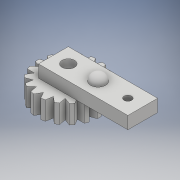
# Autodesk Inventor part: Parcial3
Saved by Autodesk Inventor 2018 (Build 220112000, 112)
## iProperties
Created: 2020-06-26
Part Number: Parcial3
Material: Generic
Document SubType Name: Modeling
Designer: Ivan
Density: 1 g/cm^3
Appearance: Default
Author: Ivan
Autodesk Inventor part; units mm, degrees
ref_plane "YZ Plane" through (0, 0, 0) normal (1, 0, 0) x (0, 1, 0)
ref_plane "XZ Plane" through (0, 0, 0) normal (0, 1, 0) x (-1, 0, 0)
ref_plane "XY Plane" through (0, 0, 0) normal (0, 0, 1) x (1, 0, 0)
sketch "Sketch1" plane through (0, 0, 0) normal (0, 0, 1) x (1, 0, 0)
  circle A0 centre (0, 0) radius 25
  circle A1 centre (0, 0) radius 5
  dimension "d0" = 50
  dimension "d1" = 10
  constraints: 2 centre point, 2 coincident
  measures "d0" diameter of A0
  measures "d1" diameter of A1
extrude "Extrusion1" add sketch "Sketch1" along normal blind 15
sketch "Sketch2" plane through (0, 0, 15) normal (0, 0, 1) x (1, 0, 0)
  circle A0 centre (0, 0) radius 25 projected
  line L0 (0, 25) -> (5, 25) construction
  line L1 (0, 20) -> (2.7962, 24.8431)
  line L2 (0, 20) -> (6.1776, 20) construction
  line L3 (0, 20) -> (-2.7962, 24.8431)
  arc A1 (2.7962, 24.8431) -> (-2.7962, 24.8431) centre (0, 0) ccw
  dimension "d5" = 5
  dimension "d7" = 60
  constraints: 8 end point, 6 point on circle, 2 horizontal, 1 centre point, 1 point on line
  measures "d5" distance of L0.start L1.start
  measures "d7" angle of L2 L1
extrude "Extrusion2" cut sketch "Sketch2" against normal through all contours L1 L3 A0 picked at (1.2433, 23.2752)
pattern_circular "Circular Pattern1" count 18 over 360 about axis through (0, 0, -10) along (0, 0, 1) of "Extrusion2"
sketch "Sketch3" plane through (0, 0, 15) normal (0, 0, 1) x (1, 0, 0)
  line L0 (-12, 12) -> (60, 12)
  line L1 (60, 12) -> (60, -12)
  line L2 (60, -12) -> (-12, -12)
  line L3 (-12, -12) -> (-12, 12)
  circle A0 centre (0, 0) radius 5 projected
  point P0 (-12, 0)
  dimension "d13" = 12
  dimension "d14" = 12
  dimension "d15" = 60
  constraints: 8 end point, 2 parallel, 1 horizontal, 1 horizontal alignment, 1 midpoint, 1 perpendicular
  measures "d13" distance from line of L3 point (0, 0)
  measures "d14" distance from line of L0 point (0, 0)
  measures "d15" distance from line of L1 point (0, 0)
extrude "Extrusion4" add sketch "Sketch3" along normal blind 10
sketch "Sketch4" plane through (0, 0, 15) normal (0, 0, -1) x (-1, 0, 0)
  circle A0 centre (-48, 0) radius 6
  line L0 (-60, 12) -> (-60, -12) construction
  point P0 (0, 0)
  dimension "d20" = 12
  dimension "d21" = 12
  constraints: 1 centre point, 1 horizontal alignment
  measures "d20" diameter of A0
  measures "d21" distance from line of L0 A0.centre
sketch "Sketch5" plane through (0, 0, 25) normal (0, 0, 1) x (1, 0, 0)
  circle A0 centre (48, 0) radius 3
  line L0 (60, -12) -> (60, 12) construction
  point P0 (0, 0)
  point P1 (0, 0)
  dimension "d22" = 6
  dimension "d23" = 12
  constraints: 1 centre point, 1 horizontal alignment
  measures "d22" diameter of A0
  measures "d23" distance from line of L0 A0.centre
loft "Loft1" cut profiles "Sketch5", "Sketch4"
sketch "Sketch6" plane through (0, 0, 25) normal (0, 0, 1) x (1, 0, 0)
  arc A0 (24, -6) -> (24, 6) centre (24, 0) ccw
  line L0 (-12, -12) -> (60, -12) projected
  line L1 (24, -6) -> (24, 6)
  point P0 (0, 0)
  point P1 (24, -12)
  dimension "d28" = 12
  constraints: 2 end point, 2 point on circle, 1 centre point, 1 horizontal alignment, 1 midpoint, 1 vertical, 1 vertical alignment
  measures "d28" diameter of A0
revolve "Revolution1" add sketch "Sketch6" angle 360 about axis through (24, -6, 25) along (0, 1, 0)
equation "\"d1\" = 0.2 * d0"
equation "\"d21\" = d20"
equation "\"d22\" = 0.5 * d20"
equation "\"d23\" = d21"
body "Solid1"
